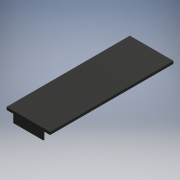
# Autodesk Inventor part: TYLNA CZARNA OBUDOWA STOJAKA
Saved by Autodesk Inventor 2017 SP1 (Build 210196100, 196)
## iProperties
Created: 2020-12-26
Part Number: TYLNA CZARNA OBUDOWA STOJAKA
Material: Tworzywo sztuczne, nieprzezroczyste czarne
Document SubType Name: Modeling
Designer: Napoleon
Mass: 19.6064 g
Surface Area: 282.43 cm^2
Volume: 20.595 cm^3
Density: 0.952 g/cm^3
Appearance: Chropowaty, teksturowany - czarny
Author: Napoleon
Autodesk Inventor part; units mm, degrees
ref_plane "YZ Plane" through (0, 0, 0) normal (1, 0, 0) x (0, 1, 0)
ref_plane "XZ Plane" through (0, 0, 0) normal (0, 1, 0) x (-1, 0, 0)
sketch "Szkic1" plane through (0, 0, 0) normal (0, 0, 1) x (1, 0, 0)
  line L0 (12.425, 226.5) -> (77.425, 226.5)
  line L1 (77.425, 226.5) -> (77.425, 42.5)
  line L2 (77.425, 42.5) -> (12.425, 42.5)
  line L3 (12.425, 42.5) -> (12.425, 226.5)
  constraints: 8 end point, 2 parallel, 1 horizontal, 1 perpendicular
extrude "Wyciągnięcie proste1" add sketch "Szkic1" along normal blind 4
shell "Skorupa1" thickness 1.5 removed faces 1 at (55.7583, 103.8333, 0)
ref_plane "Płaszczyzna konstrukcyjna1" through (20.925, 15, -12) normal (0, 0, -1) x (0, 1, 0)
sketch "Szkic2" plane through (0, 0, 0) normal (0, 0, -1) x (-1, 0, 0)
  line L0 (-13.925, 44) -> (-75.925, 44)
  line L1 (-77.425, 42.5) -> (-12.425, 42.5)
  line L2 (-22.425, 17.5) -> (-22.425, 215.5)
  arc A0 (-23.425, 16.5) -> (-22.425, 17.5) centre (-23.425, 17.5) ccw
  line L3 (-66.425, 16.5) -> (-23.425, 16.5)
  arc A1 (-67.425, 17.5) -> (-66.425, 16.5) centre (-66.425, 17.5) ccw
  line L4 (-67.425, 215.5) -> (-67.425, 17.5)
  arc A2 (-66.425, 216.5) -> (-67.425, 215.5) centre (-66.425, 215.5) ccw
  line L5 (-23.425, 216.5) -> (-66.425, 216.5)
  arc A3 (-22.425, 215.5) -> (-23.425, 216.5) centre (-23.425, 215.5) ccw
  line L6 (-20.925, 218) -> (-20.925, 15)
  line L7 (-68.925, 218) -> (-20.925, 218)
  line L8 (-68.925, 15) -> (-68.925, 218)
  line L9 (-20.925, 15) -> (-68.925, 15)
  line L10 (-1.5, 236.5) -> (-88.35, 236.5)
  line L11 (-88.35, 0) -> (-88.35, 236.5)
  line L12 (-88.35, 0) -> (-1.5, 0)
  line L13 (-1.5, 0) -> (-1.5, 236.5)
  line L14 (-68.925, 15) -> (-68.925, 218)
  line L15 (-68.925, 218) -> (-20.925, 218)
  line L16 (-20.925, 218) -> (-20.925, 15)
  line L17 (-20.925, 15) -> (-68.925, 15)
  line L18 (-22.425, 17.5) -> (-22.425, 215.5)
  arc A4 (-23.425, 16.5) -> (-22.425, 17.5) centre (-23.425, 17.5) ccw
  line L19 (-66.425, 16.5) -> (-23.425, 16.5)
  arc A5 (-67.425, 17.5) -> (-66.425, 16.5) centre (-66.425, 17.5) ccw
  line L20 (-67.425, 215.5) -> (-67.425, 17.5)
  arc A6 (-66.425, 216.5) -> (-67.425, 215.5) centre (-66.425, 215.5) ccw
  line L21 (-23.425, 216.5) -> (-66.425, 216.5)
  arc A7 (-22.425, 215.5) -> (-23.425, 216.5) centre (-23.425, 215.5) ccw
  line L22 (-20.925, 218) -> (-20.925, 15)
  line L23 (-68.925, 218) -> (-20.925, 218)
  line L24 (-68.925, 15) -> (-68.925, 218)
  line L25 (-20.925, 15) -> (-68.925, 15)
  line L26 (-68.925, 15) -> (-68.925, 218)
  line L27 (-1.5, 236.5) -> (-88.35, 236.5)
  line L28 (-88.35, 0) -> (-88.35, 236.5)
  line L29 (-88.35, 0) -> (-1.5, 0)
  line L30 (-1.5, 0) -> (-1.5, 236.5)
  line L31 (-68.925, 15) -> (-68.925, 218)
  line L32 (-68.925, 218) -> (-20.925, 218)
  line L33 (-20.925, 218) -> (-20.925, 15)
  line L34 (-20.925, 15) -> (-68.925, 15)
  line L35 (-67.425, 44) -> (-22.425, 44)
  line L36 (-22.425, 44) -> (-22.425, 42.5)
  line L37 (-22.425, 42.5) -> (-67.425, 42.5)
  line L38 (-67.425, 42.5) -> (-67.425, 44)
  point P0 (0, 0)
extrude "Wyciągnięcie proste2" add sketch "Szkic2" along normal up to surface (12 mm away) contours L2 L1 L4 L0
